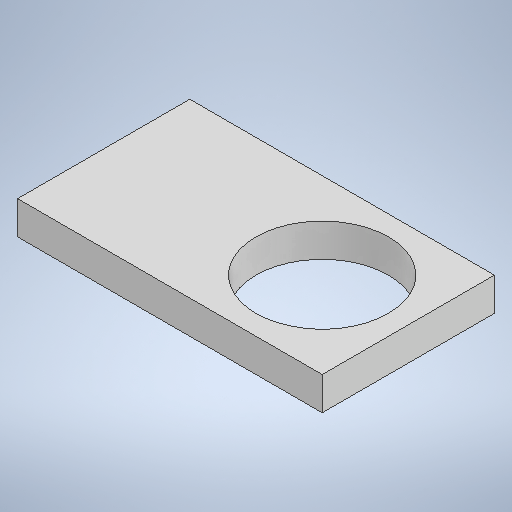
# Autodesk Inventor part: joystick_test_v1
Saved by Autodesk Inventor 2025.4 (Build 294407000, 407)
## iProperties
Created: 2026-07-26
Part Number: joystick_test_v1
Material: Generic
Document SubType Name: Modeling
Designer: Franchesca
Density: 1 g/cm^3
Appearance: Default
Author: Franchesca
Autodesk Inventor part; units mm, degrees
ref_plane "YZ Plane" through (0, 0, 0) normal (1, 0, 0) x (0, 1, 0)
ref_plane "XZ Plane" through (0, 0, 0) normal (0, 1, 0) x (-1, 0, 0)
ref_plane "XY Plane" through (0, 0, 0) normal (0, 0, 1) x (1, 0, 0)
sketch "Sketch1" plane through (0, 0, 0) normal (0, 1, 0) x (-1, 0, 0)
  circle A0 centre (0, 0) radius 10
  line L0 (0, -10) -> (30, -10) construction
  line L1 (0, 10) -> (30, 10) construction
  line L2 (30, 10) -> (30, -10) construction
  line L3 (0, -10) -> (15, -10) construction
  line L4 (0, 10) -> (15, 10) construction
  line L5 (15, 10) -> (15, -10) construction
  line L6 (30, 10) -> (30, 5) construction
  line L7 (30, -10) -> (30, -5) construction
  line L8 (30, -5) -> (30, 5)
  line L9 (30, 5) -> (15, 5)
  line L10 (30, -5) -> (15, -5)
  line L11 (15, -5) -> (15, 5)
  line L12 (0, -10) -> (0, -13) construction
  line L13 (0, 10) -> (0, 13) construction
  line L14 (30, 0) -> (33, 0) construction
  line L15 (-10, 0) -> (-13, 0) construction
  line L16 (33, 0) -> (33, -13)
  line L17 (33, -13) -> (0, -13)
  line L18 (33, 0) -> (33, 13)
  line L19 (33, 13) -> (0, 13)
  line L20 (0, 13) -> (-13, 13)
  line L21 (-13, 0) -> (-13, 13)
  line L22 (0, -13) -> (-13, -13)
  line L23 (-13, -13) -> (-13, 0)
  dimension "d0" = 20
  dimension "d1" = 30
  dimension "d2" = 30
  dimension "d3" = 15
  dimension "d4" = 15
  dimension "d5" = 5
  dimension "d6" = 5
  dimension "d7" = 3
  dimension "d8" = 3
  dimension "d9" = 3
  dimension "d10" = 3
  constraints: 48 end point, 7 point on line, 5 perpendicular, 4 horizontal, 4 vertical, 3 midpoint, 3 point on circle, 2 tangent, 1 centre point, 1 coincident, 1 collinear, 1 parallel
  measures "d0" diameter of A0
  measures "d1" distance of L0.start L0.end
  measures "d2" distance of L1.start L1.end
  measures "d3" distance of L0.start L3.end
  measures "d4" distance of L1.start L4.end
  measures "d5" distance of L1.end L6.end
  measures "d6" distance of L0.end L7.end
  measures "d7" distance of L0.start L12.end
  measures "d8" distance of L1.start L13.end
  measures "d9" distance of L14.start L14.end
  measures "d10" distance of L15.start L15.end
extrude "Extrusion1" add sketch "Sketch1" against normal blind 5
extrude "Extrusion2" add sketch "Sketch1" against normal blind 2 contours L10 L11 L9 L8
body "Solid1"
